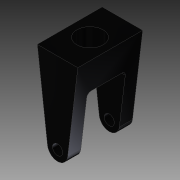
# Autodesk Inventor part: hinge_for_swing
Saved by Autodesk Inventor 2015 (Build 190159000, 159)
## iProperties
Created: 2017-02-21
Part Number: hinge_for_swing
Material: Acetal Resin, Black
Document SubType Name: Modeling
Designer: Guy
Density: 1.425 g/cm^3
Appearance: Smooth - Black
Author: Guy
Autodesk Inventor part; units mm, degrees
ref_plane "YZ Plane" through (0, 0, 0) normal (1, 0, 0) x (0, 1, 0)
ref_plane "XZ Plane" through (0, 0, 0) normal (0, 1, 0) x (-1, 0, 0)
ref_plane "XY Plane" through (0, 0, 0) normal (0, 0, 1) x (1, 0, 0)
sketch "Sketch1" plane through (0, 0, 0) normal (0, 0, 1) x (1, 0, 0)
  line L0 (0, 0) -> (5.038, 40.6155)
  circle A0 centre (10, 40) radius 5
  line L1 (14.962, 40.6155) -> (20, 0)
  line L2 (20, 0) -> (0, 0)
  circle A1 centre (10, 40) radius 2.5
  line L3 (2.5, 0) -> (2.5, 20.1545)
  line L4 (17.5, 0) -> (17.5, 20.1545)
  dimension "d0" = 5
  dimension "d1" = 10
  dimension "d2" = 20
  dimension "d3" = 10
  dimension "d4" = 40
  dimension "d19" = 15
  dimension "d20" = 7.5
  constraints: 10 end point, 4 point on line, 2 centre point, 2 point on circle, 2 tangent, 1 coincident, 1 horizontal, 1 parallel, 1 perpendicular
  measures "d0" diameter of A1
  measures "d1" diameter of A0
  measures "d2" distance of L1.end L0.start
  measures "d3" horizontal distance of L0.start A0.centre
  measures "d4" distance from line of L2 A0.centre
  measures "d19" distance between parallel lines of L3 L4
  measures "d20" distance from line of A0.centre L4
extrude "Extrusion1" add sketch "Sketch1" along normal blind 32
ref_plane "Work Plane1" through (0, 0, 16) normal (0, 0, 1) x (1, 0, 0)
sketch "Sketch2" plane through (0, 0, 16) normal (0, 0, 1) x (1, 0, 0)
  circle A0 centre (10, 40) radius 2.5 projected
  arc A1 (14.962, 40.6155) -> (5.038, 40.6155) centre (10, 40) ccw projected
  line L0 (20, 0) -> (14.962, 40.6155) projected
  line L1 (0, 0) -> (20, 0) projected
  line L2 (5.038, 40.6155) -> (0, 0) projected
  line L3 (1.8606, 52.4259) -> (18.1394, 52.4259)
  line L4 (18.1394, 52.4259) -> (18.1394, 15)
  line L5 (18.1394, 15) -> (1.8606, 15)
  line L6 (1.8606, 15) -> (1.8606, 52.4259)
  dimension "d21" = 25
  constraints: 8 end point, 2 parallel, 2 point on line, 1 horizontal, 1 perpendicular
  measures "d21" distance from line of A0.centre L5
extrude "Extrusion2" cut sketch "Sketch2" along normal mid plane 19 contours A0 | L0 L5 L2 A1 | A1 L2 L6 L3 L4 L0
sketch "Sketch3" plane through (0, 0, 0) normal (0, -1, 0) x (1, 0, 0)
  line L0 (0, 0) -> (20, 0) projected
  line L1 (20, 0) -> (20, 32) projected
  line L2 (0, 32) -> (20, 32) projected
  line L3 (0, 0) -> (0, 32) projected
  circle A0 centre (10, 16) radius 6.45
  dimension "d14" = 12.9
  dimension "d15" = 10
  dimension "d16" = 16
  constraints: 1 centre point
  measures "d14" diameter of A0
  measures "d15" distance from line of L1 A0.centre
  measures "d16" distance from line of A0.centre L2
extrude "Extrusion3" cut sketch "Sketch3" against normal up to next contours A0
fillet "Fillet1" radius 2 2 edges at (10, 15, 6.5) (10, 15, 25.5)
body "Solid1"
